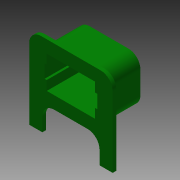
# Autodesk Inventor part: Switch Holder
Saved by Autodesk Inventor 2014 (Build 180170000, 170)
## iProperties
Created: 2016-02-05
Part Number: Switch Holder
Material: Generic
Document SubType Name: Modeling
Designer: Paul
Density: 1 g/cm^3
Appearance: Dark Green
Author: Paul
Autodesk Inventor part; units mm, degrees
ref_plane "YZ Plane" through (0, 0, 0) normal (1, 0, 0) x (0, 1, 0)
ref_plane "XZ Plane" through (0, 0, 0) normal (0, 1, 0) x (-1, 0, 0)
ref_plane "XY Plane" through (0, 0, 0) normal (0, 0, 1) x (1, 0, 0)
sketch "Sketch1" plane through (0, 0, 0) normal (0, 1, 0) x (-1, 0, 0)
  line L0 (-10.1425, -6.7516) -> (10.1425, -6.7516)
  line L1 (10.1425, -6.7516) -> (10.1425, 6.7516)
  line L2 (10.1425, 6.7516) -> (-10.1425, 6.7516)
  line L3 (-10.1425, 6.7516) -> (-10.1425, -6.7516)
  line L4 (-10.1425, -6.7516) -> (10.1425, 6.7516) construction
  line L5 (10.1425, -6.7516) -> (-10.1425, 6.7516) construction
  line L6 (-13.125, -9.7516) -> (13.125, -9.7516)
  line L7 (13.125, -9.7516) -> (13.125, 9.7516)
  line L8 (13.125, 9.7516) -> (-13.125, 9.7516)
  line L9 (-13.125, 9.7516) -> (-13.125, -9.7516)
  point P0 (0, 0)
  point P1 (0, 0)
  point P2 (0, 0)
  point P3 (0, -9.7516)
  point P4 (0, 0)
  point P5 (-13.125, 0)
  point P6 (0, 0)
  dimension "d2" = 19.685
  dimension "d3" = 12.9032
  dimension "d4" = 3
  dimension "d12" = 26.25
  constraints: 20 end point, 8 midpoint, 4 parallel, 2 horizontal, 2 perpendicular, 1 coincident, 1 horizontal alignment, 1 vertical alignment
  measures "d4" distance between parallel lines of L6 L0
  measures "d12" distance between parallel lines of L7 L9
extrude "Extrusion1" add sketch "Sketch1" along normal blind 18
sketch "Sketch2" plane through (0, 0, 0) normal (0, -1, 0) x (1, 0, 0)
  line L0 (10.1425, 6.7516) -> (10.1425, -6.7516) projected
  line L1 (10.1425, -6.7516) -> (-10.1425, -6.7516) projected
  line L2 (-10.1425, -6.7516) -> (-10.1425, 6.7516) projected
  line L3 (-10.1425, 6.7516) -> (10.1425, 6.7516) projected
  line L4 (17.5, -22.7) -> (17.5, 12)
  line L5 (17.5, 12) -> (-17.5, 12)
  line L6 (-17.5, 12) -> (-17.5, -22.7)
  line L7 (13.125, -9.7516) -> (-13.125, -9.7516) projected
  line L8 (-13.125, 9.7516) -> (13.125, 9.7516) projected
  line L9 (-13.125, -9.7516) -> (-13.125, 9.7516) projected
  line L10 (-12, -22.7) -> (-12, -17)
  line L11 (-7, -12) -> (7, -12)
  line L12 (12, -17) -> (12, -22.7)
  line L13 (0, -23.1968) -> (0, 12) construction
  line L14 (-17.5, -22.7) -> (-12, -22.7)
  line L15 (12, -22.7) -> (17.5, -22.7)
  arc A0 (-7, -12) -> (-12, -17) centre (-7, -17) ccw
  arc A1 (12, -17) -> (7, -12) centre (7, -17) ccw
  point P0 (0, 0)
  point P1 (0, 0)
  point P2 (-12, -12)
  point P3 (12, -12)
  dimension "d8" = 35
  dimension "d13" = 12
  dimension "d15" = 2.2484
  dimension "d16" = 2.2484
  dimension "d17" = 22.7
  dimension "d18" = 24
  dimension "d32" = 34.7
  dimension "d33" = 5
  constraints: 18 end point, 6 parallel, 5 perpendicular, 4 point on circle, 4 point on line, 4 tangent, 2 centre point, 2 horizontal, 1 coincident, 1 equal radius, 1 midpoint, 1 vertical alignment, 1 other
  measures "d8" distance of L4.end L5.end
  measures "d13" distance from line of L5 point (0, 0)
  measures "d15" distance between parallel lines of L7 L11
  measures "d16" distance between parallel lines of L5 L8
  measures "d17" distance from line of point (0, 0) L14
  measures "d18" distance between parallel lines of L10 L12
  measures "d32" distance between parallel lines of L14 L5
  measures "d33" radius of A0
extrude "Extrusion2" add sketch "Sketch2" against normal blind 1.5
sketch "Sketch3" plane through (0, 0, 0) normal (0, 0, 1) x (1, 0, 0)
  line L0 (-13.125, 1.5) -> (-13.125, 18) projected
  line L1 (13.125, 18) -> (-13.125, 18) projected
  line L2 (-10.1425, 0) -> (-10.1425, 18) projected
  line L3 (10.1425, 0) -> (10.1425, 18) projected
  line L4 (13.125, 1.5) -> (13.125, 18) projected
  line L5 (7, 0) -> (-7, 0) projected
  line L6 (-11.05, 0) -> (-11.05, 14.5925)
  line L7 (-11.05, 14.5925) -> (-10.1425, 15.5)
  line L8 (11.05, 0) -> (11.05, 14.5925)
  line L9 (11.05, 14.5925) -> (10.1425, 15.5)
  line L10 (0, 18) -> (0, 0) construction
  line L11 (-10.1425, 17.0925) -> (-11.05, 18)
  line L12 (-11.05, 14.5925) -> (-11.05, 18) construction
  line L13 (10.1425, 17.0925) -> (11.05, 18)
  line L14 (11.05, 18) -> (11.05, 14.5925) construction
  line L15 (-10.1425, 0) -> (-11.05, 0)
  line L16 (10.1425, 0) -> (11.05, 0)
  line L17 (-10.1425, 15.5) -> (-10.1425, 0)
  line L18 (10.1425, 0) -> (10.1425, 15.5)
  line L19 (10.1425, 17.0925) -> (10.1425, 18)
  line L20 (10.1425, 18) -> (11.05, 18)
  line L21 (-11.05, 18) -> (-10.1425, 18)
  line L22 (-10.1425, 18) -> (-10.1425, 17.0925)
  dimension "d21" = 2.5
  dimension "d22" = 21.5
  dimension "d24" = 45
  dimension "d34" = 20.285
  constraints: 34 end point, 8 point on line, 4 collinear, 4 parallel, 4 perpendicular, 2 vertical, 1 horizontal alignment, 1 midpoint, 2 other
  measures "d21" distance of L2.end L7.end
  measures "d24" angle of L8 L9
  measures "d34" distance of L2.start L3.start
extrude "Extrusion3" cut sketch "Sketch3" along normal mid plane 5.6
fillet "Fillet1" radius 5 2 edges at (17.5, 0.75, 12) (-17.5, 0.75, 12)
fillet "Fillet2" radius 5 4 edges at (13.125, 9.75, 9.7516) (13.125, 9.75, -9.7516) (-13.125, 9.75, 9.7516) (-13.125, 9.75, -9.7516)
equation "\"d15\" = d16"
body "Solid1"
